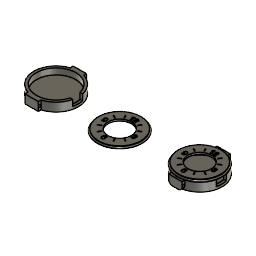
LockClock (Autodesk Fusion 360 design; units mm, degrees)
Autodesk Fusion 360 part; units mm, degrees
(part 1 of 3)
sketch "Esboço1" plane through (0, 0, 0) normal (0, 0, 1) x (1, 0, 0)
  circle A0 centre (-25, 20) radius 15.5
  circle A1 centre (-25, 20) radius 17.5
  line L0 (-30.5466, 36.597748) -> (-20, 36.597748)
  line L1 (-20, 36.597748) -> (-20, 39.000001)
  line L2 (-20, 39.000001) -> (-30.5466, 39.000001)
  line L3 (-30.5466, 39.000001) -> (-30.5466, 36.597748)
  line L4 (-30.5466, 3.402252) -> (-30.5466, 0.999999)
  line L5 (-20, 3.402252) -> (-30.5466, 3.402252)
  line L6 (-20, 0.999999) -> (-20, 3.402252)
  line L7 (-30.5466, 0.999999) -> (-20, 0.999999)
  dimension "d1" = 31
  dimension "d2" = 35
  dimension "d3" = 16.597748
  dimension "d4" = 16.597748
  constraint concentric A0 A1
  constraint horizontal L0
  constraint vertical L1
  constraint horizontal L2
  constraint vertical L3
  constraint horizontal L7
  constraint vertical L6
  constraint horizontal L5
  constraint vertical L4
  measures "d1" diameter of A0
  measures "d2" diameter of A1
  measures "d3" distance of A0.centre L0
  measures "d4" distance of A0.centre L5
extrude "Extrusão1" add sketch "Esboço1" along normal blind 2 contours A0 picked at (-21.496516, 20.274828) makes body 1
extrude "Extrusão2" add sketch "Esboço1" along normal blind 6.8 contours A1 L0 L1 L5 L6 picked at (-41.801896, 20) bodies 1
extrude "Extrusão3" add sketch "Esboço1" along normal blind 6.8 contours A1 L1 L2 L3 | A1 L0 L1 | A1 L5 L6 | A1 L4 L6 L7 picked at (-24.920681, 38.494135) picked at (-26.341436, 36.782153) picked at (-26.341436, 3.217847) picked at (-24.920681, 1.505865) bodies 1
hole "Furo1" at (-20, 37.885255, 3.4) direction (-1, 0, 0) diameter 2 depth 10.5 tip angle 118 bodies 1
hole "Furo2" at (-20, 2.114745, 3.4) direction (-1, 0, 0) diameter 2 depth 10.5 tip angle 118 bodies 1
sketch "Esboço2" plane through (0, 0, 6.8) normal (0, 0, 1) x (-1, 0, 0)
  circle A0 centre (25, -20) radius 15.5
  arc A1 (20, -3.22949) -> (20, -36.77051) centre (25, -20) ccw
  line L0 (20, -36.77051) -> (20, -39.000001)
  line L1 (20, -39.000001) -> (30.5466, -39.000001)
  line L2 (30.5466, -39.000001) -> (30.5466, -36.597748)
  arc A2 (30.5466, -36.597748) -> (30.5466, -3.402252) centre (25, -20) ccw
  line L3 (30.5466, -3.402252) -> (30.5466, -0.999999)
  line L4 (30.5466, -0.999999) -> (20, -0.999999)
  line L5 (20, -0.999999) -> (20, -3.22949)
  line L6 (9.949815, -23.707012) -> (7, -23.707012)
  line L7 (7, -23.707012) -> (7, -16)
  line L8 (7, -16) -> (9.949815, -16)
  line L9 (9.949815, -16) -> (9.949815, -23.707012)
  constraint horizontal L6
  constraint vertical L7
  constraint horizontal L8
  constraint vertical L9
extrude "Extrusão4" cut sketch "Esboço2" against normal blind 4.7 contours A0 A1 L6 L8 L9 picked at (8.199032, -19.900154) bodies 1
sketch "Esboço3" plane through (0, 0, 0) normal (0, 0, 1) x (1, 0, 0)
  circle A0 centre (25, 20) radius 17.5
  circle A1 centre (25, 20) radius 9.225
  dimension "d19" = 35
  dimension "d20" = 18.45
  constraint concentric A0 A1
  measures "d19" diameter of A0
  measures "d20" diameter of A1
extrude "Extrusão5" add sketch "Esboço3" along normal blind 1 separate body makes body 2
fillet "Arredondamento1" radius 0.9 1 edges at (8.684272, 13.67173, 1) on bodies 2
sketch "Esboço4" plane through (0, 0, 1) normal (0, 0, 1) x (-1, 0, 0)
  circle A0 centre (-25, -20) radius 9.225
  circle A1 centre (-25, -20) radius 16.6
  spline S0 degree 3 poles (-24.643786, -36.277315) (-33.480346, -36.277315) (-40.643786, -29.113875) (-40.643786, -20.277315) (-40.643786, -20.277315) (-40.643786, -11.440755) (-33.480346, -4.277315) (-24.643786, -4.277315) (-24.643786, -4.277315) (-15.807226, -4.277315) (-8.643786, -11.440755) (-8.643786, -20.277315) (-8.643786, -20.277315) (-8.643786, -29.113875) (-15.807226, -36.277315) (-24.643786, -36.277315) knots 0 0 0 0 0.2 0.2 0.2 0.20000001 0.4 0.4 0.4 0.40000001 0.6 0.6 0.6 0.60000001 1 1 1 1
  line L0 (-22.930276, -30.044155) -> (-22.930276, -32.475195)
  line L1 (-22.930276, -32.475195) -> (-22.080936, -32.475195)
  line L2 (-22.080936, -32.475195) -> (-22.080936, -32.973615)
  line L3 (-22.080936, -32.973615) -> (-22.136036, -32.973615)
  spline S1 degree 3 poles (-22.136036, -32.973615) (-22.136237, -32.973626) (-22.13664, -32.97361) (-22.137445, -32.973618) (-22.138853, -32.973614) (-22.140862, -32.973619) (-22.14327, -32.973623) (-22.146475, -32.973633) (-22.150472, -32.973649) (-22.156845, -32.973686) (-22.164777, -32.973751) (-22.174254, -32.973861) (-22.183677, -32.974002) (-22.196132, -32.974232) (-22.211564, -32.974597) (-22.229918, -32.975162) (-22.253956, -32.976077) (-22.283462, -32.977529) (-22.318207, -32.979784) (-22.352078, -32.98254) (-22.385075, -32.985796) (-22.427376, -32.990744) (-22.47811, -32.998126) (-22.536294, -33.009098) (-22.590999, -33.022066) (-22.657572, -33.04152) (-22.732789, -33.07046) (-22.787796, -33.10102) (-22.812456, -33.117705) knots 0 0 0 0 0.00006041 0.00012081 0.00024154 0.00048274 0.00072359 0.00096411 0.00144412 0.00192277 0.00287599 0.00382377 0.00476614 0.00570309 0.00756081 0.00939703 0.01121183 0.0147776 0.01825895 0.02165679 0.02497206 0.0282058 0.03443289 0.04034821 0.04596329 0.05129156 0.06114811 0.07008033 0.07008033 0.07008033 0.07008033
  spline S2 degree 3 poles (-22.812456, -33.117705) (-22.812536, -33.117782) (-22.812737, -33.117885) (-22.813097, -33.118146) (-22.813747, -33.118577) (-22.814662, -33.119207) (-22.815763, -33.119961) (-22.817226, -33.120972) (-22.819049, -33.122241) (-22.821228, -33.123775) (-22.823397, -33.125319) (-22.826276, -33.127392) (-22.82985, -33.13001) (-22.834103, -33.133195) (-22.83972, -33.137496) (-22.846648, -33.142979) (-22.854813, -33.149731) (-22.862825, -33.156653) (-22.870685, -33.163744) (-22.880966, -33.173429) (-22.893447, -33.185969) (-22.907807, -33.201685) (-22.92156, -33.218079) (-22.939161, -33.240936) (-22.959672, -33.271291) (-22.981726, -33.310241) (-23.001341, -33.35187) (-23.018522, -33.396168) (-23.033276, -33.443128) (-23.050057, -33.510638) (-23.05844, -33.56326) (-23.062506, -33.599175) knots 0 0 0 0 0.00003338 0.00006676 0.00013351 0.00026697 0.00040039 0.00053376 0.00080037 0.0010668 0.00133308 0.0015992 0.002131 0.00266226 0.00319305 0.00425345 0.00531268 0.00637124 0.00742961 0.00848828 0.01060834 0.01273539 0.01487326 0.01702569 0.02138789 0.02585092 0.03044079 0.03518129 0.04009386 0.04519765 0.05604103 0.05604103 0.05604103 0.05604103
  line L4 (-23.062506, -33.599175) -> (-23.632126, -33.599175)
  line L5 (-23.632126, -33.599175) -> (-23.632126, -30.044155)
  line L6 (-23.632126, -30.044155) -> (-22.930276, -30.044155)
  spline S3 degree 3 poles (-24.678956, -30.044155) (-24.682356, -30.362025) (-24.750166, -30.631575) (-24.883246, -30.852805) knots 0 0 0 0 0.04545455 0.04545455 0.04545455 0.04545455
  spline S4 degree 3 poles (-24.883246, -30.852805) (-24.883346, -30.852939) (-24.883497, -30.85324) (-24.883853, -30.853807) (-24.884451, -30.854816) (-24.885321, -30.856249) (-24.886363, -30.857972) (-24.887762, -30.86027) (-24.889519, -30.863142) (-24.892356, -30.867741) (-24.895944, -30.873492) (-24.900312, -30.880387) (-24.904747, -30.887284) (-24.910765, -30.896505) (-24.918456, -30.908037) (-24.927934, -30.921852) (-24.93768, -30.935675) (-24.947696, -30.949507) (-24.961476, -30.968053) (-24.979383, -30.991257) (-25.001843, -31.019002) (-25.025377, -31.046782) (-25.058519, -31.084241) (-25.102702, -31.131144) (-25.159491, -31.187014) (-25.220566, -31.24302) (-25.285922, -31.299164) (-25.355558, -31.355447) (-25.455978, -31.432101) (-25.534951, -31.487622) (-25.589326, -31.524145) knots 0 0 0 0 0.0000502 0.00010042 0.0002009 0.00040204 0.0006034 0.000805 0.00120888 0.00161369 0.00242612 0.00324231 0.00406232 0.00488616 0.00654552 0.00822069 0.00991195 0.01161956 0.01334379 0.01684307 0.02041179 0.02405178 0.02776476 0.03541574 0.04337698 0.05165893 0.06027084 0.0692209 0.07851635 0.09816704 0.09816704 0.09816704 0.09816704
  spline S5 degree 3 poles (-25.589326, -31.524145) (-25.590403, -31.524864) (-25.592551, -31.526354) (-25.596957, -31.529338) (-25.605009, -31.534797) (-25.61704, -31.542867) (-25.632227, -31.552956) (-25.654426, -31.567564) (-25.684651, -31.587192) (-25.723929, -31.612322) (-25.767161, -31.63962) (-25.797352, -31.658457) (-25.813106, -31.668235) knots 0 0 0 0 0.00038853 0.00078416 0.00159668 0.00330677 0.00513014 0.00706667 0.01127873 0.01594193 0.02105522 0.02661755 0.02661755 0.02661755 0.02661755
  spline S6 degree 3 poles (-25.813106, -31.668235) (-25.813169, -31.668294) (-25.813328, -31.668369) (-25.813613, -31.668565) (-25.814127, -31.668885) (-25.814852, -31.669355) (-25.815725, -31.669913) (-25.816888, -31.670659) (-25.81834, -31.671591) (-25.820659, -31.673082) (-25.823552, -31.674946) (-25.827017, -31.677183) (-25.830473, -31.679419) (-25.835064, -31.682397) (-25.84078, -31.686119) (-25.847609, -31.690588) (-25.856648, -31.696532) (-25.867857, -31.703958) (-25.881188, -31.712879) (-25.894373, -31.721793) (-25.907413, -31.730699) (-25.924537, -31.742518) (-25.94558, -31.757273) (-25.97035, -31.775021) (-25.994538, -31.79274) (-26.025754, -31.816135) (-26.063339, -31.845297) (-26.106491, -31.880472) (-26.147315, -31.915533) (-26.18581, -31.95048) (-26.221978, -31.985315) (-26.266316, -32.030812) (-26.316193, -32.087386) (-26.367857, -32.156118) (-26.410228, -32.224483) (-26.443279, -32.292496) (-26.463237, -32.34954) (-26.474284, -32.394732) (-26.480144, -32.42815) (-26.483077, -32.455973) (-26.484256, -32.478131) (-26.484538, -32.495691) (-26.484279, -32.514115) (-26.483314, -32.53948) (-26.480885, -32.570353) (-26.475974, -32.606324) (-26.466905, -32.651856) (-26.450695, -32.705785) (-26.422964, -32.765801) (-26.387227, -32.820279) (-26.35839, -32.85257) (-26.342886, -32.867655) knots 0 0 0 0 0.00002593 0.00005188 0.00010375 0.00020747 0.00031114 0.00041476 0.00062185 0.00082874 0.00124193 0.00165433 0.00206594 0.00247676 0.00329604 0.00411217 0.00492516 0.00654171 0.00814575 0.00973729 0.01131638 0.01288306 0.0159793 0.01902634 0.0220245 0.02497413 0.03072918 0.03629467 0.04167407 0.04687118 0.05189025 0.05673598 0.06592736 0.07449569 0.08250156 0.0900192 0.09713812 0.10058218 0.10396727 0.10730869 0.10896823 0.11062286 0.11257612 0.1144954 0.11823741 0.12186133 0.12538037 0.13215824 0.13870058 0.14514542 0.15163497 0.15163497 0.15163497 0.15163497
  spline S7 degree 3 poles (-26.342886, -32.867655) (-26.342848, -32.867675) (-26.342796, -32.867748) (-26.342667, -32.867859) (-26.342454, -32.86807) (-26.342143, -32.868362) (-26.341772, -32.868716) (-26.341276, -32.869186) (-26.340655, -32.869773) (-26.339659, -32.870709) (-26.338412, -32.871875) (-26.336909, -32.873266) (-26.335401, -32.87465) (-26.333383, -32.876486) (-26.330846, -32.878762) (-26.32778, -32.881465) (-26.323663, -32.885029) (-26.318461, -32.889411) (-26.312129, -32.894554) (-26.305708, -32.899579) (-26.299198, -32.904487) (-26.290398, -32.910876) (-26.27917, -32.918573) (-26.265345, -32.927336) (-26.251165, -32.935628) (-26.231722, -32.946089) (-26.206471, -32.957996) (-26.174844, -32.970338) (-26.141788, -32.980781) (-26.107303, -32.989322) (-26.071387, -32.99596) (-26.020753, -33.002376) (-25.953126, -33.005431) (-25.871201, -33.001346) (-25.79126, -32.987572) (-25.718031, -32.964284) (-25.651616, -32.931398) (-25.592188, -32.888923) (-25.557742, -32.854679) (-25.541866, -32.836295) knots 0 0 0 0 0.00001282 0.00002564 0.00005128 0.00010256 0.00015384 0.0002051 0.00030762 0.00041011 0.00061501 0.00081982 0.00102455 0.00122918 0.00163821 0.00204695 0.00245542 0.0032717 0.00408733 0.00490258 0.0057177 0.00653297 0.00816493 0.00980066 0.01144228 0.01309189 0.01642285 0.01981024 0.02326956 0.02681543 0.03046151 0.03422045 0.04211996 0.05073603 0.05878133 0.06638717 0.07370922 0.08092219 0.08820933 0.08820933 0.08820933 0.08820933
  spline S8 degree 3 poles (-25.541866, -32.836295) (-25.541814, -32.836213) (-25.54167, -32.83608) (-25.541425, -32.835783) (-25.540976, -32.835276) (-25.540347, -32.834543) (-25.539589, -32.833664) (-25.538584, -32.832489) (-25.537331, -32.831016) (-25.535337, -32.828649) (-25.532864, -32.82567) (-25.52993, -32.822065) (-25.527028, -32.818429) (-25.523198, -32.813538) (-25.518491, -32.807345) (-25.512974, -32.799793) (-25.505776, -32.789543) (-25.497094, -32.776412) (-25.487206, -32.760184) (-25.477829, -32.74346) (-25.468962, -32.72624) (-25.45775, -32.702467) (-25.445017, -32.671438) (-25.43188, -32.632454) (-25.420783, -32.591481) (-25.408478, -32.533138) (-25.398446, -32.454869) (-25.396066, -32.390673) (-25.396066, -32.357375) knots 0 0 0 0 0.00002898 0.00005797 0.00011594 0.0002319 0.00034787 0.00046386 0.00069589 0.00092799 0.00139244 0.00185724 0.00232245 0.00278809 0.00372088 0.00465596 0.00559366 0.00747819 0.00937722 0.01129332 0.01322902 0.01518675 0.01917713 0.02328288 0.02752039 0.03190456 0.04116254 0.05115198 0.05115198 0.05115198 0.05115198
  line L7 (-25.396066, -32.357375) -> (-25.396066, -32.327705)
  line L8 (-25.396066, -32.327705) -> (-24.739996, -32.327705)
  spline S9 degree 3 poles (-24.739996, -32.327705) (-24.740008, -32.327837) (-24.73999, -32.328103) (-24.739999, -32.328634) (-24.739994, -32.329562) (-24.739999, -32.330888) (-24.74, -32.332478) (-24.740006, -32.334597) (-24.740015, -32.337242) (-24.740036, -32.341469) (-24.740073, -32.346743) (-24.740135, -32.35306) (-24.740215, -32.359362) (-24.740345, -32.367734) (-24.740553, -32.37816) (-24.740873, -32.390626) (-24.741393, -32.407126) (-24.742221, -32.4276) (-24.743501, -32.451982) (-24.745066, -32.476118) (-24.746915, -32.50001) (-24.749748, -32.531396) (-24.753992, -32.570029) (-24.760247, -32.615622) (-24.767643, -32.660236) (-24.778931, -32.717947) (-24.795842, -32.787768) (-24.820878, -32.86833) (-24.850497, -32.944986) (-24.884703, -33.017727) (-24.923499, -33.086547) (-24.966886, -33.15144) (-25.014857, -33.212393) (-25.049839, -33.250338) (-25.068026, -33.268595) knots 0 0 0 0 0.0000398 0.00007961 0.00015921 0.00031833 0.00047736 0.00063629 0.00095386 0.00127106 0.00190431 0.00253604 0.00316626 0.00379498 0.00504791 0.00629488 0.00753594 0.01000044 0.0124418 0.01486036 0.0172565 0.01963061 0.02431419 0.02891448 0.03343495 0.03787924 0.0465538 0.05497215 0.06317041 0.07118772 0.07906588 0.08684895 0.09458261 0.10231343 0.10231343 0.10231343 0.10231343
  spline S10 degree 3 poles (-25.068026, -33.268595) (-25.06807, -33.268618) (-25.068128, -33.268708) (-25.068277, -33.268843) (-25.068522, -33.269099) (-25.068881, -33.269455) (-25.069308, -33.269885) (-25.069879, -33.270457) (-25.070593, -33.271173) (-25.071736, -33.272315) (-25.073168, -33.273741) (-25.074889, -33.275447) (-25.076615, -33.277148) (-25.07892, -33.279411) (-25.081812, -33.282228) (-25.085296, -33.28559) (-25.089962, -33.29005) (-25.095832, -33.295579) (-25.102938, -33.302143) (-25.110103, -33.308636) (-25.117329, -33.315057) (-25.127043, -33.323522) (-25.139338, -33.333926) (-25.154334, -33.346123) (-25.16957, -33.358034) (-25.19022, -33.373543) (-25.216653, -33.392221) (-25.249314, -33.413468) (-25.282941, -33.433566) (-25.317533, -33.452514) (-25.353091, -33.470312) (-25.402053, -33.49263) (-25.465823, -33.517648) (-25.545779, -33.542883) (-25.629593, -33.563505) (-25.717262, -33.579517) (-25.808789, -33.590923) (-25.887531, -33.596545) (-25.95239, -33.5988) (-26.015394, -33.59953) (-26.091039, -33.597859) (-26.205163, -33.589722) (-26.340997, -33.569528) (-26.494454, -33.52806) (-26.635799, -33.469656) (-26.764834, -33.394316) (-26.842312, -33.333003) (-26.878596, -33.299955) knots 0 0 0 0 0.00001515 0.00003031 0.00006063 0.00012127 0.0001819 0.00024253 0.00036378 0.00048501 0.00072744 0.00096983 0.00121216 0.00145445 0.00193889 0.00242317 0.00290729 0.00387509 0.00484241 0.00580931 0.00677591 0.00774229 0.00967472 0.01160737 0.01354096 0.01547621 0.01935446 0.02324807 0.02716277 0.03110417 0.03507779 0.03908903 0.04724388 0.05560997 0.06422431 0.07312088 0.08233055 0.0918812 0.09679269 0.10179858 0.11078234 0.11948215 0.13611229 0.15189242 0.1670539 0.18185688 0.19658031 0.19658031 0.19658031 0.19658031
  spline S11 degree 3 poles (-26.878596, -33.299955) (-26.87862, -33.299914) (-26.878707, -33.299862) (-26.878842, -33.299726) (-26.879096, -33.299503) (-26.879449, -33.299176) (-26.879876, -33.298787) (-26.880444, -33.298268) (-26.881153, -33.297618) (-26.882287, -33.296577) (-26.883701, -33.295275) (-26.885394, -33.293709) (-26.887083, -33.292141) (-26.889328, -33.290047) (-26.892122, -33.287423) (-26.895459, -33.284262) (-26.899882, -33.280035) (-26.905367, -33.274725) (-26.911881, -33.268306) (-26.918324, -33.261844) (-26.924695, -33.255339) (-26.933088, -33.246617) (-26.943402, -33.235606) (-26.955507, -33.222207) (-26.967326, -33.208636) (-26.982686, -33.190336) (-27.001186, -33.167019) (-27.022274, -33.138313) (-27.042222, -33.108917) (-27.06103, -33.078831) (-27.078697, -33.048055) (-27.100767, -33.006035) (-27.125542, -32.951655) (-27.150631, -32.883761) (-27.171138, -32.813113) (-27.187064, -32.73972) (-27.198413, -32.663585) (-27.205186, -32.584708) (-27.207689, -32.492612) (-27.203673, -32.389716) (-27.18957, -32.278832) (-27.165869, -32.173125) (-27.132518, -32.072619) (-27.089494, -31.977359) (-27.054421, -31.917499) (-27.035406, -31.888625) knots 0 0 0 0 0.00001444 0.00002888 0.00005777 0.00011553 0.00017328 0.00023102 0.00034648 0.00046191 0.00069265 0.00092324 0.00115369 0.001384 0.00184419 0.00230383 0.00276292 0.00367949 0.00459397 0.00550645 0.00641697 0.00732563 0.00913761 0.01094298 0.01274234 0.01453627 0.01811016 0.02166966 0.02521971 0.02876529 0.0323114 0.03586301 0.04300139 0.05022079 0.05755907 0.06505224 0.07273417 0.08063628 0.08878746 0.10036033 0.1114921 0.12227448 0.13280897 0.14320498 0.15357696 0.15357696 0.15357696 0.15357696
  spline S12 degree 3 poles (-27.035406, -31.888625) (-27.035319, -31.88852) (-27.035187, -31.888282) (-27.03488, -31.887835) (-27.034362, -31.887038) (-27.033608, -31.885907) (-27.032704, -31.884546) (-27.03149, -31.88273) (-27.029963, -31.880457) (-27.027493, -31.876811) (-27.024362, -31.872243) (-27.020542, -31.866757) (-27.016653, -31.861255) (-27.011354, -31.853868) (-27.004555, -31.844595) (-26.99615, -31.833447) (-26.987468, -31.822236) (-26.978507, -31.810962) (-26.966095, -31.795728) (-26.949874, -31.77653) (-26.929445, -31.753413) (-26.907906, -31.730045) (-26.877268, -31.698095) (-26.836132, -31.657558) (-26.783028, -31.608595) (-26.725498, -31.558645) (-26.663547, -31.507712) (-26.597174, -31.455801) (-26.500574, -31.383641) (-26.424779, -31.330587) (-26.372556, -31.295275) knots 0 0 0 0 0.00004064 0.00008131 0.00016271 0.00032574 0.0004891 0.00065278 0.00098112 0.00131076 0.00197396 0.00264244 0.00331621 0.0039953 0.00536961 0.0067656 0.00818352 0.00962357 0.01108597 0.01407858 0.01716288 0.02034023 0.02361188 0.03044219 0.03766203 0.045278 0.05329567 0.06171973 0.07055417 0.08946649 0.08946649 0.08946649 0.08946649
  spline S13 degree 3 poles (-26.372556, -31.295275) (-26.371823, -31.294779) (-26.370372, -31.293752) (-26.367425, -31.29172) (-26.362179, -31.288088) (-26.35453, -31.282833) (-26.345137, -31.276417) (-26.332065, -31.267544) (-26.315025, -31.256076) (-26.28593, -31.236684) (-26.246791, -31.210931) (-26.196502, -31.178242) (-26.141883, -31.143056) (-26.104004, -31.118808) (-26.084356, -31.106255) knots 0 0 0 0 0.00026552 0.00053303 0.00107399 0.00217973 0.00331719 0.00448632 0.00691952 0.00947905 0.01497598 0.02097474 0.02747277 0.03446748 0.03446748 0.03446748 0.03446748
  spline S14 degree 3 poles (-26.084356, -31.106255) (-26.08396, -31.105981) (-26.083137, -31.10548) (-26.081527, -31.10443) (-26.078701, -31.102619) (-26.074684, -31.100023) (-26.069878, -31.096918) (-26.063512, -31.092794) (-26.055609, -31.087659) (-26.043107, -31.079501) (-26.027699, -31.069381) (-26.009484, -31.057312) (-25.991622, -31.045366) (-25.968473, -31.029738) (-25.940412, -31.010518) (-25.907849, -30.987746) (-25.867088, -30.958601) (-25.819614, -30.923456) (-25.767133, -30.882425) (-25.720294, -30.843389) (-25.6791, -30.806353) (-25.643551, -30.771313) (-25.613644, -30.738269) (-25.589371, -30.707201) (-25.570728, -30.678097) (-25.561452, -30.658699) (-25.557966, -30.649375) knots 0 0 0 0 0.0001444 0.00028866 0.00057677 0.00115128 0.00172353 0.00229352 0.00342671 0.00455086 0.00677202 0.00895704 0.01110593 0.01321873 0.01733612 0.02130949 0.02513912 0.03236847 0.03902775 0.04512167 0.05065669 0.05564178 0.06008962 0.06401851 0.06745554 0.07044179 0.07044179 0.07044179 0.07044179
  line L9 (-25.557966, -30.649375) -> (-27.171876, -30.649375)
  line L10 (-27.171876, -30.649375) -> (-27.171876, -30.044155)
  line L11 (-27.171876, -30.044155) -> (-24.678956, -30.044155)
  line L12 (-34.911586, -19.636505) -> (-35.593096, -19.636505)
  spline S15 degree 3 poles (-35.593096, -19.636505) (-35.593108, -19.636376) (-35.593094, -19.636116) (-35.593106, -19.635598) (-35.59311, -19.634691) (-35.593126, -19.633397) (-35.593143, -19.631846) (-35.59317, -19.629782) (-35.593208, -19.627206) (-35.593278, -19.623099) (-35.593385, -19.617984) (-35.593544, -19.611871) (-35.593733, -19.60579) (-35.594026, -19.597746) (-35.594466, -19.58777) (-35.595117, -19.575895) (-35.596141, -19.560314) (-35.59772, -19.541153) (-35.600109, -19.518555) (-35.602981, -19.49647) (-35.606337, -19.474899) (-35.611408, -19.447093) (-35.618923, -19.413569) (-35.629963, -19.375001) (-35.64294, -19.338488) (-35.662548, -19.293179) (-35.691932, -19.24112) (-35.721366, -19.204082) (-35.737196, -19.187255) knots 0 0 0 0 0.00003889 0.00007778 0.00015552 0.00031086 0.00046599 0.00062093 0.00093021 0.00123871 0.00185334 0.00246484 0.00307322 0.0036785 0.00487983 0.00606895 0.00724599 0.00956438 0.01183616 0.01406258 0.01624491 0.01838455 0.02254128 0.02654589 0.03041269 0.03415754 0.04134779 0.0482784 0.0482784 0.0482784 0.0482784
  spline S16 degree 3 poles (-35.737196, -19.187255) (-35.737235, -19.187234) (-35.737284, -19.187151) (-35.737414, -19.187028) (-35.737627, -19.186794) (-35.737939, -19.186469) (-35.73831, -19.186075) (-35.738807, -19.185552) (-35.739428, -19.1849) (-35.740426, -19.183859) (-35.741677, -19.182563) (-35.743186, -19.181016) (-35.744702, -19.179477) (-35.746733, -19.177436) (-35.74929, -19.174906) (-35.752389, -19.171903) (-35.756558, -19.167943) (-35.761845, -19.163075) (-35.768306, -19.157365) (-35.774885, -19.151787) (-35.781581, -19.146342) (-35.790673, -19.139252) (-35.802341, -19.130714) (-35.8168, -19.121008) (-35.83173, -19.111829) (-35.852363, -19.100241) (-35.879409, -19.087066) (-35.913587, -19.073457) (-35.949648, -19.061963) (-35.987593, -19.052578) (-36.027425, -19.045297) (-36.084182, -19.03825) (-36.156635, -19.035141) (-36.241771, -19.038682) (-36.32151, -19.050124) (-36.394541, -19.069488) (-36.460818, -19.096871) (-36.520223, -19.132338) (-36.555189, -19.161421) (-36.571276, -19.177085) knots 0 0 0 0 0.00001352 0.00002705 0.0000541 0.0001082 0.00016229 0.00021638 0.00032453 0.00043266 0.00064885 0.00086496 0.00108099 0.00129695 0.00172867 0.00216017 0.00259148 0.00345376 0.00431588 0.00517821 0.00604113 0.00690499 0.00863693 0.01037703 0.01212816 0.01389314 0.01747489 0.02114397 0.02491992 0.02882069 0.03286254 0.03706009 0.04597041 0.0545823 0.06259068 0.07008862 0.07719074 0.08403312 0.09076916 0.09076916 0.09076916 0.09076916
  spline S17 degree 3 poles (-36.571276, -19.177085) (-36.571296, -19.177124) (-36.571376, -19.177172) (-36.571495, -19.1773) (-36.571722, -19.177509) (-36.572036, -19.177815) (-36.572416, -19.178179) (-36.572921, -19.178667) (-36.573552, -19.179277) (-36.574557, -19.180257) (-36.57581, -19.181485) (-36.577305, -19.182965) (-36.578792, -19.184452) (-36.580764, -19.186444) (-36.583209, -19.188951) (-36.586111, -19.191986) (-36.589938, -19.196069) (-36.594642, -19.20124) (-36.600159, -19.207555) (-36.605549, -19.213978) (-36.610812, -19.220509) (-36.617661, -19.229365) (-36.625909, -19.240713) (-36.635288, -19.254754) (-36.644157, -19.269225) (-36.655348, -19.289176) (-36.66807, -19.315259) (-36.681222, -19.348136) (-36.69233, -19.382721) (-36.7014, -19.41901) (-36.708437, -19.456997) (-36.713448, -19.496679) (-36.716425, -19.538055) (-36.717416, -19.580544) (-36.71633, -19.623019) (-36.711724, -19.677105) (-36.700295, -19.740851) (-36.676639, -19.811746) (-36.643207, -19.875542) (-36.600012, -19.932036) (-36.5653, -19.964238) (-36.546696, -19.978955) knots 0 0 0 0 0.00001317 0.00002634 0.00005268 0.00010537 0.00015804 0.00021071 0.00031603 0.00042132 0.00063183 0.00084224 0.00105256 0.0012628 0.00168304 0.002103 0.00252272 0.0033616 0.00420004 0.00503836 0.0058769 0.00671599 0.00839705 0.01008428 0.01178025 0.01348754 0.01694533 0.02047744 0.02410172 0.02783465 0.03169119 0.03568487 0.03982776 0.04413061 0.04843063 0.05256736 0.060408 0.06779699 0.07490281 0.08191509 0.08903164 0.08903164 0.08903164 0.08903164
  spline S18 degree 3 poles (-36.546696, -19.978955) (-36.546652, -19.978973) (-36.546589, -19.979049) (-36.546437, -19.979158) (-36.546183, -19.97937) (-36.545813, -19.979662) (-36.545372, -19.980016) (-36.544782, -19.980486) (-36.544043, -19.981073) (-36.542858, -19.982009) (-36.541371, -19.983175) (-36.539577, -19.984566) (-36.537775, -19.985949) (-36.535358, -19.987785) (-36.532313, -19.990061) (-36.528626, -19.992761) (-36.523655, -19.996327) (-36.517348, -20.000709) (-36.509645, -20.005842) (-36.501796, -20.010856) (-36.493802, -20.015751) (-36.482911, -20.022142) (-36.468924, -20.029833) (-36.451619, -20.038553) (-36.433734, -20.046799) (-36.415269, -20.054569) (-36.396225, -20.061864) (-36.369807, -20.071048) (-36.335277, -20.081315) (-36.291932, -20.091622) (-36.246285, -20.100038) (-36.198339, -20.106569) (-36.156914, -20.110402) (-36.122651, -20.112561) (-36.096109, -20.113725) (-36.073631, -20.11431) (-36.055363, -20.114528) (-36.043992, -20.11461) (-36.034739, -20.114522) (-36.024189, -20.1142) (-36.008526, -20.113422) (-35.995346, -20.112551) (-35.988096, -20.112035) knots 0 0 0 0 0.00001413 0.00002826 0.00005652 0.00011306 0.00016962 0.00022619 0.00033939 0.00045264 0.00067934 0.00090631 0.00113353 0.00136103 0.00181687 0.00227386 0.00273205 0.00365219 0.00457767 0.00550883 0.00644602 0.00738955 0.00929692 0.01123353 0.01320181 0.01520403 0.01724238 0.01931889 0.0235936 0.02804279 0.03267892 0.03751294 0.04255441 0.04515573 0.04781196 0.05052398 0.05190119 0.05329265 0.0539352 0.054677 0.05645902 0.05863958 0.05863958 0.05863958 0.05863958
  spline S19 degree 3 poles (-35.988096, -20.112035) (-35.986159, -20.111909) (-35.98237, -20.111625) (-35.975119, -20.111148) (-35.963875, -20.110449) (-35.949868, -20.109753) (-35.939312, -20.109485) (-35.934696, -20.109485) knots 0 0 0 0 0.00058232 0.00113975 0.00217996 0.00396198 0.00534694 0.00534694 0.00534694 0.00534694
  line L13 (-35.934696, -20.109485) -> (-35.934696, -20.602815)
  line L14 (-35.934696, -20.602815) -> (-36.011836, -20.602815)
  spline S20 degree 3 poles (-36.011836, -20.602815) (-36.012102, -20.602834) (-36.012637, -20.602807) (-36.013703, -20.602821) (-36.015567, -20.602815) (-36.018225, -20.602828) (-36.021409, -20.602843) (-36.025636, -20.602873) (-36.030898, -20.602927) (-36.03926, -20.603048) (-36.049625, -20.603263) (-36.061959, -20.603626) (-36.074155, -20.604093) (-36.090141, -20.604849) (-36.109782, -20.606051) (-36.132928, -20.607917) (-36.162717, -20.610928) (-36.198607, -20.615699) (-36.239964, -20.623162) (-36.27912, -20.632304) (-36.31608, -20.64313) (-36.361557, -20.659499) (-36.413503, -20.684094) (-36.45095, -20.70945) (-36.467866, -20.723185) knots 0 0 0 0 0.00008009 0.00016013 0.00032006 0.00063926 0.00095759 0.00127506 0.0019074 0.00253631 0.00378383 0.00501773 0.00623811 0.00744506 0.00981909 0.01214075 0.01441099 0.01880104 0.02299849 0.02701362 0.03085817 0.03454548 0.04150636 0.04804324 0.04804324 0.04804324 0.04804324
  spline S21 degree 3 poles (-36.467866, -20.723185) (-36.467887, -20.72322) (-36.467966, -20.723259) (-36.468087, -20.723371) (-36.468315, -20.72355) (-36.468632, -20.723815) (-36.469016, -20.72413) (-36.469525, -20.724552) (-36.470161, -20.725079) (-36.471176, -20.725926) (-36.472439, -20.726989) (-36.473947, -20.728271) (-36.475448, -20.72956) (-36.477437, -20.731288) (-36.479903, -20.733464) (-36.482832, -20.736105) (-36.486692, -20.73966) (-36.491438, -20.744175) (-36.497008, -20.749705) (-36.50245, -20.755346) (-36.507765, -20.761097) (-36.51468, -20.768913) (-36.52301, -20.778967) (-36.532492, -20.791472) (-36.541461, -20.80442) (-36.552777, -20.82234) (-36.565658, -20.84592) (-36.578987, -20.87587) (-36.590251, -20.907582) (-36.599453, -20.941052) (-36.606595, -20.976278) (-36.611684, -21.013261) (-36.61471, -21.051999) (-36.61551, -21.084093) (-36.615217, -21.108826) (-36.613557, -21.151674) (-36.606156, -21.20856) (-36.585623, -21.276269) (-36.561075, -21.328871) (-36.529338, -21.376683) (-36.503703, -21.405005) (-36.489906, -21.418245) knots 0 0 0 0 0.00001241 0.00002482 0.00004963 0.00009926 0.00014887 0.00019847 0.00029765 0.00039678 0.00059491 0.00079287 0.00099068 0.00118833 0.00158319 0.0019775 0.00237131 0.00315756 0.00394233 0.00472598 0.00550887 0.00629135 0.00785651 0.00942445 0.01099809 0.01258028 0.01578091 0.01904887 0.02240466 0.02586722 0.02945381 0.03317996 0.03705952 0.04110477 0.04280641 0.04447918 0.05397023 0.05990311 0.0656453 0.0713206 0.07705741 0.07705741 0.07705741 0.07705741
  spline S22 degree 3 poles (-36.489906, -21.418245) (-36.489872, -21.418262) (-36.489827, -21.418328) (-36.489713, -21.418426) (-36.489524, -21.418613) (-36.489249, -21.418873) (-36.488921, -21.419187) (-36.488482, -21.419604) (-36.487934, -21.420125) (-36.487054, -21.420956) (-36.485951, -21.421991) (-36.484623, -21.423226) (-36.48329, -21.424454) (-36.481507, -21.426083) (-36.479266, -21.428103) (-36.476556, -21.4305) (-36.472919, -21.433661) (-36.468323, -21.437545) (-36.462729, -21.442103) (-36.457058, -21.446555) (-36.451309, -21.450901) (-36.443539, -21.456556) (-36.433627, -21.463364) (-36.421423, -21.471109) (-36.408908, -21.478432) (-36.391755, -21.487661) (-36.369481, -21.498153) (-36.341587, -21.509013) (-36.312442, -21.518186) (-36.282044, -21.525675) (-36.250391, -21.531486) (-36.205777, -21.537095) (-36.146297, -21.539728) (-36.074303, -21.53629) (-36.004056, -21.52485) (-35.939555, -21.505545) (-35.880871, -21.478344) (-35.828135, -21.443261) (-35.797243, -21.414862) (-35.782966, -21.399605) knots 0 0 0 0 0.00001135 0.00002271 0.00004543 0.00009085 0.00013626 0.00018167 0.00027247 0.00036324 0.00054471 0.00072608 0.00090736 0.00108854 0.00145064 0.00181243 0.00217392 0.00289615 0.00361758 0.00433846 0.00505902 0.00577953 0.00722127 0.00866568 0.01011472 0.01157031 0.01450821 0.01749462 0.02054355 0.02366818 0.02688075 0.0301925 0.0371515 0.04471242 0.05177802 0.05845006 0.06484885 0.07111026 0.07737889 0.07737889 0.07737889 0.07737889
  spline S23 degree 3 poles (-35.782966, -21.399605) (-35.78292, -21.399537) (-35.782794, -21.399426) (-35.782578, -21.399178) (-35.782185, -21.398756) (-35.781632, -21.398145) (-35.780967, -21.397413) (-35.780083, -21.396434) (-35.778983, -21.395208) (-35.777231, -21.393236) (-35.775059, -21.390756) (-35.77248, -21.387755) (-35.769929, -21.384729) (-35.766564, -21.380661) (-35.762425, -21.375512) (-35.757571, -21.369235) (-35.75124, -21.360725) (-35.743599, -21.34983) (-35.734883, -21.336369) (-35.726612, -21.322507) (-35.718785, -21.308243) (-35.70889, -21.288584) (-35.697633, -21.262942) (-35.68599, -21.230722) (-35.67614, -21.196881) (-35.66521, -21.148764) (-35.65626, -21.0842) (-35.654126, -21.031214) (-35.654126, -21.003755) knots 0 0 0 0 0.00002472 0.00004944 0.00009889 0.00019777 0.00029666 0.00039555 0.00059332 0.0007911 0.00118669 0.00158234 0.0019781 0.002374 0.00316635 0.00395969 0.00475429 0.00634836 0.00795087 0.00956401 0.01118998 0.0128309 0.01616539 0.01958398 0.02310164 0.02673221 0.03437927 0.04261699 0.04261699 0.04261699 0.04261699
  line L15 (-35.654126, -21.003755) -> (-35.654126, -20.974085)
  line L16 (-35.654126, -20.974085) -> (-34.982796, -20.974085)
  spline S24 degree 3 poles (-34.982796, -20.974085) (-34.98281, -20.974202) (-34.982799, -20.97444) (-34.982818, -20.974913) (-34.982833, -20.975742) (-34.982864, -20.976924) (-34.982899, -20.978342) (-34.982948, -20.980232) (-34.983011, -20.982591) (-34.983118, -20.986361) (-34.983262, -20.991065) (-34.98345, -20.996699) (-34.983655, -21.002319) (-34.983948, -21.009786) (-34.984355, -21.019086) (-34.984907, -21.030204) (-34.985728, -21.044921) (-34.986913, -21.063182) (-34.988594, -21.084927) (-34.990531, -21.106453) (-34.992725, -21.12776) (-34.995978, -21.155754) (-35.000677, -21.19021) (-35.007368, -21.230863) (-35.015087, -21.27064) (-35.026659, -21.322106) (-35.043657, -21.384362) (-35.068343, -21.456129) (-35.097171, -21.524375) (-35.130143, -21.589086) (-35.167272, -21.650256) (-35.222209, -21.726944) (-35.269888, -21.779364) (-35.304046, -21.811555) knots 0 0 0 0 0.00003551 0.00007102 0.00014203 0.00028399 0.00042587 0.00056767 0.00085101 0.00113402 0.00169906 0.00226278 0.00282519 0.00338629 0.00450461 0.00561776 0.00672579 0.00892662 0.01110743 0.01326855 0.01541033 0.01753312 0.02172307 0.0258415 0.02989159 0.03387668 0.04166518 0.04923814 0.05662862 0.06387231 0.07100725 0.07807335 0.09215408 0.09215408 0.09215408 0.09215408
  spline S25 degree 3 poles (-35.304046, -21.811555) (-35.304087, -21.811575) (-35.304143, -21.811655) (-35.304283, -21.811773) (-35.304516, -21.811999) (-35.304854, -21.812312) (-35.305258, -21.812691) (-35.305798, -21.813195) (-35.306473, -21.813825) (-35.307554, -21.814832) (-35.308908, -21.816087) (-35.310536, -21.81759) (-35.312167, -21.819089) (-35.314346, -21.821082) (-35.317079, -21.823563) (-35.320373, -21.826526) (-35.324782, -21.830454) (-35.330327, -21.835326) (-35.337037, -21.841109) (-35.343801, -21.846829) (-35.35062, -21.852486) (-35.359787, -21.859946) (-35.371384, -21.869116) (-35.385517, -21.879864) (-35.399869, -21.890361) (-35.419318, -21.904036) (-35.444193, -21.920506) (-35.474888, -21.939237) (-35.506462, -21.956958) (-35.538916, -21.973668) (-35.572249, -21.989366) (-35.618137, -22.009065) (-35.67783, -22.031145) (-35.752555, -22.053417) (-35.830806, -22.071624) (-35.912586, -22.085768) (-35.9979, -22.095848) (-36.086756, -22.101868) (-36.204522, -22.104352) (-36.346388, -22.098815) (-36.50681, -22.077581) (-36.655129, -22.041728) (-36.79131, -21.991137) (-36.915228, -21.92573) (-36.98991, -21.871962) (-37.024766, -21.842915) knots 0 0 0 0 0.00001384 0.00002769 0.00005539 0.00011079 0.00016619 0.00022158 0.00033237 0.00044316 0.00066471 0.00088625 0.00110777 0.00132928 0.00177226 0.00221521 0.00265811 0.00354388 0.00442963 0.00531546 0.00620144 0.00708765 0.00886106 0.01063634 0.01241412 0.01419502 0.01776854 0.02136201 0.02498032 0.02862824 0.03231046 0.03603154 0.0436068 0.0513888 0.05940871 0.06769515 0.07627419 0.08516944 0.09440216 0.11160327 0.12770634 0.14287023 0.15728558 0.17117466 0.18478631 0.18478631 0.18478631 0.18478631
  spline S26 degree 3 poles (-37.024766, -21.842915) (-37.02479, -21.842878) (-37.024872, -21.842834) (-37.025001, -21.842715) (-37.025242, -21.842521) (-37.025579, -21.842236) (-37.025986, -21.841896) (-37.026528, -21.841443) (-37.027204, -21.840876) (-37.028285, -21.839969) (-37.029634, -21.838832) (-37.031248, -21.837466) (-37.032858, -21.836098) (-37.034998, -21.834271) (-37.037663, -21.83198) (-37.040845, -21.829221) (-37.045061, -21.825532) (-37.05029, -21.820896) (-37.056501, -21.81529) (-37.062644, -21.809644) (-37.06872, -21.803959) (-37.076719, -21.796337) (-37.086551, -21.78671) (-37.098092, -21.774985) (-37.109363, -21.763104) (-37.123999, -21.747084) (-37.141629, -21.726656) (-37.161739, -21.701466) (-37.180761, -21.675644) (-37.198696, -21.649192) (-37.215544, -21.622109) (-37.236571, -21.585131) (-37.260188, -21.537202) (-37.284126, -21.47721) (-37.30369, -21.414689) (-37.318882, -21.349644) (-37.329706, -21.282078) (-37.335052, -21.224126) (-37.337187, -21.176585) (-37.337754, -21.139612) (-37.337071, -21.102063) (-37.334851, -21.064417) (-37.331154, -21.027546) (-37.32429, -20.979756) (-37.312031, -20.921744) (-37.291226, -20.854749) (-37.264429, -20.790872) (-37.242591, -20.750417) (-37.230746, -20.730815) knots 0 0 0 0 0.00001324 0.0000265 0.000053 0.000106 0.00015898 0.00021196 0.00031788 0.00042376 0.00063539 0.00084686 0.00105816 0.0012693 0.00169109 0.00211223 0.00253274 0.00337188 0.00420857 0.00504289 0.0058749 0.00670466 0.00835772 0.01000264 0.01163999 0.01327033 0.01651219 0.01973307 0.02293778 0.0261312 0.02931829 0.032504 0.03888998 0.04532993 0.05186245 0.05852455 0.06535118 0.07237488 0.0759705 0.07962638 0.08346624 0.08723426 0.0909366 0.09457981 0.10171462 0.10869859 0.11559378 0.12246462 0.12246462 0.12246462 0.12246462
  spline S27 degree 3 poles (-37.230746, -20.730815) (-37.230638, -20.730673) (-37.230474, -20.730354) (-37.230092, -20.729752) (-37.229447, -20.728683) (-37.228509, -20.727166) (-37.227383, -20.725346) (-37.225872, -20.722924) (-37.223969, -20.719905) (-37.220893, -20.715092) (-37.21699, -20.709108) (-37.212215, -20.701982) (-37.207347, -20.694908) (-37.200728, -20.685542) (-37.19222, -20.673964) (-37.181647, -20.660292) (-37.170703, -20.646832) (-37.159388, -20.633584) (-37.143764, -20.616155) (-37.123281, -20.594886) (-37.097287, -20.570287) (-37.06981, -20.546538) (-37.030839, -20.515727) (-36.978214, -20.479332) (-36.933551, -20.453353) (-36.910336, -20.440915) knots 0 0 0 0 0.00005349 0.00010699 0.00021399 0.000428 0.00064204 0.0008561 0.0012843 0.00171263 0.00256971 0.00342748 0.00428608 0.00514563 0.00686809 0.00859594 0.01033022 0.01207196 0.01382215 0.01735166 0.02092678 0.02455499 0.02824345 0.03582645 0.04372773 0.04372773 0.04372773 0.04372773
  spline S28 degree 3 poles (-36.910336, -20.440915) (-36.910564, -20.440793) (-36.911051, -20.440612) (-36.911993, -20.440183) (-36.91318, -20.43967) (-36.914598, -20.439042) (-36.916488, -20.438207) (-36.918845, -20.43716) (-36.922605, -20.435479) (-36.927288, -20.433365) (-36.932883, -20.430807) (-36.938449, -20.428231) (-36.945821, -20.424774) (-36.954965, -20.420405) (-36.965839, -20.415077) (-36.980144, -20.40789) (-36.997741, -20.398712) (-37.018458, -20.387358) (-37.038713, -20.375693) (-37.058507, -20.363716) (-37.084163, -20.347408) (-37.115115, -20.326239) (-37.150581, -20.299461) (-37.184194, -20.271423) (-37.226319, -20.232555) (-37.27459, -20.180624) (-37.30843, -20.135368) (-37.323986, -20.112035) knots 0 0 0 0 0.00007767 0.00015532 0.00031054 0.00046564 0.00062062 0.00093025 0.00123941 0.00185637 0.00247152 0.00308486 0.00369642 0.00491423 0.00612506 0.00732904 0.00971687 0.01207873 0.01441563 0.01672864 0.01901884 0.02353507 0.02797407 0.03234586 0.03666101 0.04516304 0.05357591 0.05357591 0.05357591 0.05357591
  spline S29 degree 3 poles (-37.323986, -20.112035) (-37.324006, -20.111984) (-37.324082, -20.111901) (-37.324197, -20.111715) (-37.324416, -20.111398) (-37.324719, -20.110941) (-37.325086, -20.110395) (-37.325574, -20.109665) (-37.326182, -20.108752) (-37.327153, -20.10729) (-37.328362, -20.10546) (-37.329806, -20.103259) (-37.331241, -20.101053) (-37.333144, -20.098107) (-37.335504, -20.094414) (-37.338306, -20.089963) (-37.341999, -20.084006) (-37.34654, -20.076516) (-37.351865, -20.067455) (-37.357067, -20.058324) (-37.362145, -20.049123) (-37.368754, -20.036756) (-37.376709, -20.021117) (-37.385759, -20.002073) (-37.394316, -19.982746) (-37.40509, -19.956549) (-37.417335, -19.923054) (-37.430027, -19.881815) (-37.440754, -19.839446) (-37.452543, -19.780938) (-37.460247, -19.720571) (-37.463572, -19.666728) (-37.46454, -19.635108) (-37.464824, -19.604409) (-37.464294, -19.567196) (-37.461899, -19.509835) (-37.455908, -19.439937) (-37.44378, -19.358435) (-37.421343, -19.254972) (-37.38111, -19.132119) (-37.312387, -18.99551) (-37.223814, -18.871463) (-37.15279, -18.798424) (-37.114616, -18.764275) knots 0 0 0 0 0.00001646 0.00003292 0.00006584 0.00013168 0.00019752 0.00026336 0.00039501 0.00052666 0.0007899 0.00105308 0.00131621 0.00157929 0.00210532 0.00263118 0.0031569 0.00420802 0.00525888 0.00630966 0.00736057 0.0084118 0.01051595 0.0126237 0.01473659 0.01685614 0.02112087 0.02543004 0.02979507 0.03422687 0.04332946 0.04802173 0.05040683 0.0528192 0.05723133 0.06157009 0.07004104 0.07826381 0.08627207 0.10178321 0.11690214 0.13197181 0.14733752 0.14733752 0.14733752 0.14733752
  spline S30 degree 3 poles (-37.114616, -18.764275) (-37.11457, -18.764253) (-37.114505, -18.764168) (-37.114347, -18.764041) (-37.114084, -18.763798) (-37.113701, -18.763462) (-37.113244, -18.763054) (-37.112634, -18.762513) (-37.11187, -18.761836) (-37.110648, -18.760755) (-37.109118, -18.759406) (-37.107278, -18.757792) (-37.105435, -18.756182) (-37.102972, -18.754041) (-37.099886, -18.751376) (-37.096168, -18.748194) (-37.091193, -18.743974) (-37.08494, -18.738742) (-37.07738, -18.732531) (-37.069766, -18.726388) (-37.062096, -18.720313) (-37.051794, -18.712302) (-37.038778, -18.702457) (-37.022939, -18.690916) (-37.00688, -18.679646) (-36.985154, -18.66497) (-36.957429, -18.647296) (-36.923306, -18.627195) (-36.8883, -18.608182) (-36.852412, -18.590257) (-36.815639, -18.573419) (-36.765173, -18.552309) (-36.699753, -18.528652) (-36.618141, -18.504779) (-36.533008, -18.485267) (-36.444356, -18.470114) (-36.352188, -18.459316) (-36.2565, -18.452868) (-36.127466, -18.450145) (-35.970749, -18.456527) (-35.792932, -18.481401) (-35.630111, -18.523396) (-35.482342, -18.582636) (-35.349808, -18.65918) (-35.271472, -18.721983) (-35.235386, -18.755805) knots 0 0 0 0 0.00001529 0.00003059 0.0000612 0.0001224 0.00018361 0.00024481 0.00036722 0.00048961 0.00073439 0.00097915 0.00122388 0.0014686 0.00195799 0.00244731 0.00293658 0.00391502 0.00489336 0.0058717 0.00685012 0.00782868 0.00978655 0.01174596 0.01370753 0.01567189 0.01961126 0.02356913 0.02755036 0.03155968 0.03560176 0.03968113 0.04796825 0.0564559 0.06517545 0.07415589 0.08342374 0.09300312 0.10291589 0.12213374 0.13998884 0.15668165 0.17245627 0.18760047 0.20243797 0.20243797 0.20243797 0.20243797
  spline S31 degree 3 poles (-35.235386, -18.755805) (-35.235326, -18.755881) (-35.23517, -18.755998) (-35.234896, -18.756269) (-35.234399, -18.756727) (-35.2337, -18.75739) (-35.232857, -18.758182) (-35.231737, -18.759242) (-35.230339, -18.760568) (-35.228109, -18.762694) (-35.225331, -18.765361) (-35.222016, -18.768575) (-35.218718, -18.771804) (-35.214345, -18.776127) (-35.208924, -18.781565) (-35.202486, -18.788149) (-35.194001, -18.796999) (-35.183569, -18.808204) (-35.171328, -18.82188) (-35.15937, -18.835781) (-35.147694, -18.849907) (-35.1325, -18.869043) (-35.114203, -18.893541) (-35.09338, -18.92383) (-35.073688, -18.955017) (-35.048856, -18.997935) (-35.020607, -19.05397) (-34.991368, -19.124546) (-34.966659, -19.198682) (-34.946476, -19.276366) (-34.93081, -19.357591) (-34.915666, -19.472639) (-34.911586, -19.561226) (-34.911586, -19.621245) knots 0 0 0 0 0.00002892 0.00005785 0.0001157 0.00023139 0.00034706 0.00046271 0.00069395 0.00092511 0.00138721 0.00184901 0.00231053 0.00277178 0.0036935 0.00461426 0.00553415 0.00737165 0.00920671 0.01104004 0.01287235 0.01470434 0.01837 0.02204283 0.02572841 0.02943226 0.03691506 0.04453461 0.05233056 0.06033981 0.0685963 0.07713086 0.09513662 0.09513662 0.09513662 0.09513662
  line L17 (-34.911586, -19.621245) -> (-34.911586, -19.636505)
  ellipse E0 centre (-37.965337, -18.755095) end of major axis (-51.664923, -30.555593) minor radius 3.150551 (-24.112306, -7.439615) -> (-24.264886, -6.955605) ccw
  spline S32 degree 3 poles (-24.264886, -6.955605) (-24.264929, -6.955578) (-24.264981, -6.955483) (-24.265122, -6.955336) (-24.265351, -6.955059) (-24.265688, -6.954673) (-24.266089, -6.954207) (-24.266625, -6.953588) (-24.267296, -6.952815) (-24.26837, -6.951582) (-24.269718, -6.950046) (-24.271341, -6.948213) (-24.272969, -6.94639) (-24.275147, -6.943973) (-24.277884, -6.940977) (-24.281194, -6.937418) (-24.285632, -6.932731) (-24.291239, -6.926969) (-24.298069, -6.920202) (-24.304991, -6.913592) (-24.312007, -6.907138) (-24.321471, -6.898756) (-24.33354, -6.888661) (-24.348422, -6.877154) (-24.36368, -6.866272) (-24.384521, -6.8526) (-24.411586, -6.837032) (-24.445583, -6.820862) (-24.481101, -6.807199) (-24.518141, -6.79604) (-24.556707, -6.787381) (-24.596801, -6.781214) (-24.638429, -6.777543) (-24.680163, -6.776362) (-24.721001, -6.777509) (-24.772132, -6.782206) (-24.832884, -6.793941) (-24.900962, -6.818152) (-24.96306, -6.852341) (-25.019068, -6.896465) (-25.051588, -6.931634) (-25.066756, -6.950525) knots 0 0 0 0 0.00001538 0.00003076 0.00006151 0.000123 0.00018446 0.00024591 0.00036873 0.00049145 0.00073664 0.00098148 0.00122598 0.00147013 0.00195742 0.00244341 0.00292814 0.00389394 0.00485518 0.00581218 0.00676528 0.00771483 0.00960459 0.01148435 0.01335697 0.01522537 0.01896046 0.02271368 0.0265081 0.03036605 0.03430877 0.03835622 0.04252684 0.0468375 0.05087468 0.05477545 0.06223308 0.06937034 0.07636452 0.08340348 0.09067141 0.09067141 0.09067141 0.09067141
  spline S33 degree 3 poles (-25.066756, -6.950525) (-25.066774, -6.950569) (-25.066851, -6.950635) (-25.066963, -6.950791) (-25.067179, -6.951053) (-25.067476, -6.951433) (-25.067837, -6.951888) (-25.068315, -6.952495) (-25.068913, -6.953255) (-25.069867, -6.954473) (-25.071055, -6.956) (-25.072472, -6.95784) (-25.073882, -6.959688) (-25.075753, -6.962161) (-25.078073, -6.965272) (-25.080826, -6.969032) (-25.084459, -6.974089) (-25.088927, -6.980484) (-25.094165, -6.98827) (-25.099284, -6.996173) (-25.104283, -7.004194) (-25.110803, -7.015068) (-25.118656, -7.028962) (-25.127579, -7.046068) (-25.136022, -7.063644) (-25.146707, -7.087859) (-25.158854, -7.119365) (-25.171406, -7.158815) (-25.182025, -7.200148) (-25.190712, -7.243367) (-25.197462, -7.288475) (-25.202279, -7.335474) (-25.205145, -7.384369) (-25.206085, -7.433207) (-25.205139, -7.480779) (-25.202148, -7.525861) (-25.197157, -7.569191) (-25.185854, -7.636332) (-25.167779, -7.700396) (-25.137275, -7.77049) (-25.107367, -7.823594) (-25.077675, -7.861837) (-25.061676, -7.879535) knots 0 0 0 0 0.00001449 0.00002898 0.00005797 0.00011594 0.00017392 0.00023191 0.00034791 0.00046394 0.00069609 0.00092836 0.00116075 0.00139328 0.00185875 0.0023248 0.00279147 0.00372681 0.00466506 0.00560652 0.00655147 0.00750019 0.00941003 0.01133831 0.01328717 0.01525872 0.01927739 0.02341018 0.02767128 0.03207373 0.03662939 0.04134908 0.04624257 0.05131872 0.05599951 0.06051271 0.06486831 0.06907732 0.0809381 0.08469474 0.09200027 0.09915776 0.09915776 0.09915776 0.09915776
  spline S34 degree 3 poles (-25.061676, -7.879535) (-25.061635, -7.879558) (-25.061586, -7.879644) (-25.061455, -7.879773) (-25.061241, -7.88002) (-25.060926, -7.880361) (-25.060552, -7.880774) (-25.060051, -7.881323) (-25.059424, -7.882009) (-25.058419, -7.883102) (-25.057158, -7.884463) (-25.055639, -7.886089) (-25.054113, -7.887705) (-25.05207, -7.889848) (-25.049501, -7.892505) (-25.046391, -7.89566) (-25.042213, -7.899818) (-25.036924, -7.904929) (-25.03047, -7.910927) (-25.023913, -7.916787) (-25.017253, -7.922507) (-25.008238, -7.929947) (-24.996705, -7.938905) (-24.98245, -7.949104) (-24.967783, -7.958747) (-24.947633, -7.970893) (-24.921354, -7.984711) (-24.888268, -7.999023) (-24.85356, -8.011114) (-24.817239, -8.020987) (-24.779312, -8.028647) (-24.739787, -8.034102) (-24.698668, -8.037351) (-24.643301, -8.038736) (-24.575884, -8.035417) (-24.499226, -8.022437) (-24.428625, -8.000486) (-24.364203, -7.969464) (-24.306133, -7.929353) (-24.272154, -7.896955) (-24.256406, -7.879535) knots 0 0 0 0 0.00001395 0.0000279 0.00005579 0.00011157 0.00016733 0.00022308 0.00033455 0.00044596 0.00066864 0.00089112 0.00111341 0.00133552 0.0017792 0.00222221 0.00266457 0.00354755 0.00442847 0.00530767 0.00618548 0.00706225 0.00881388 0.01056534 0.0123193 0.01407842 0.01762195 0.02121707 0.02488322 0.02863861 0.0325001 0.03648303 0.04060131 0.04486739 0.05309312 0.06080827 0.06813088 0.07520083 0.08217538 0.08922034 0.08922034 0.08922034 0.08922034
  spline S35 degree 3 poles (-24.256406, -7.879535) (-24.256354, -7.879458) (-24.256214, -7.879332) (-24.255972, -7.87905) (-24.255532, -7.87857) (-24.254913, -7.877876) (-24.254169, -7.877045) (-24.253181, -7.875933) (-24.251949, -7.87454) (-24.24999, -7.872302) (-24.24756, -7.869487) (-24.244675, -7.866084) (-24.241821, -7.862653) (-24.238056, -7.858044) (-24.233427, -7.852215) (-24.227997, -7.845115) (-24.220916, -7.835499) (-24.212371, -7.823208) (-24.202622, -7.808046) (-24.19337, -7.792461) (-24.184615, -7.776451) (-24.173555, -7.754439) (-24.160973, -7.725801) (-24.147951, -7.689905) (-24.136933, -7.652318) (-24.124726, -7.599111) (-24.114712, -7.528018) (-24.112306, -7.469736) (-24.112306, -7.439615) knots 0 0 0 0 0.00002789 0.00005579 0.00011158 0.00022315 0.00033472 0.00044628 0.0006694 0.0008925 0.00133867 0.00178485 0.00223108 0.00267737 0.00357034 0.00446405 0.00535881 0.00715254 0.00895393 0.01076528 0.01258886 0.01442689 0.01815441 0.02196509 0.02587463 0.02989759 0.03833337 0.04736975 0.04736975 0.04736975 0.04736975
  ellipse E1 centre (-38.672314, 11.349327) end of major axis (-24.19589, -8.448604) minor radius 4.342708 (-24.395426, -8.554265) -> (-24.102136, -8.367785) ccw